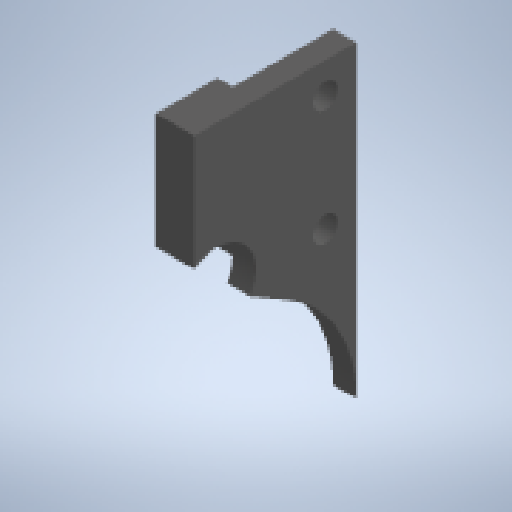
# Autodesk Inventor part: toe_springjoint_cover_upper_left
Saved by Autodesk Inventor 2024.1 (Build 281209000, 209)
## iProperties
Created: 2024-02-25
Part Number: toe_springjoint_cover_upper_left
Material: 一般
Document SubType Name: Modeling
Designer: hibik
Density: 1 g/cm^3
Appearance: 既定
Author: hibik
Autodesk Inventor part; units mm, degrees
ref_plane "YZ Plane" through (0, 0, 0) normal (1, 0, 0) x (0, 1, 0)
ref_plane "XZ Plane" through (0, 0, 0) normal (0, 1, 0) x (-1, 0, 0)
ref_plane "XY Plane" through (0, 0, 0) normal (0, 0, 1) x (1, 0, 0)
sketch "スケッチ1" plane through (0, 0, 0) normal (1, 0, 0) x (0, 1, 0)
  circle A0 centre (0, 0) radius 9
  line L0 (50, 5.5) -> (-9, 5.5)
  line L1 (-9, 5.5) -> (-9, -13.5)
  line L2 (-9, -13.5) -> (50, -13.5)
  line L3 (50, -13.5) -> (50, 5.5)
  line L4 (50, 13.5) -> (-9, 13.5)
  line L5 (-9, 13.5) -> (-9, -13.5)
  line L6 (-9, -13.5) -> (50, -13.5)
  line L7 (50, -13.5) -> (50, 13.5)
  line L8 (-20.8, 0) -> (61.8, 0) projected
  point P0 (-9, 0)
  dimension "d0" = 18
  dimension "d3" = 19
  dimension "d4" = 27
  constraints: 16 end point, 4 parallel, 2 horizontal, 2 perpendicular, 1 centre point, 1 coincident, 1 midpoint, 1 point on line, 1 tangent
  measures "d0" diameter of A0
  measures "d3" distance of L2.end L0.start
  measures "d4" distance of L4.end L1.end
extrude "押し出し1" add sketch "スケッチ1" along normal blind 1.5 contours L8 L3 L2 L1 A0 | A0 L0 L3 L8 | L1 L0 A0
sketch "スケッチ2" plane through (0, 0, 0) normal (-1, 0, 0) x (0, 0, 1)
  line L0 (1.5, 20) -> (1.5, 12.5) projected
  arc A0 (1.5, 12.5) -> (-2.1169, 9.1701) centre (0, 10.5) ccw projected
  line L1 (-2.1169, 9.1701) -> (-3.5, 8.3716) projected
  line L2 (-3.5, 8.3716) -> (-3.5, 20) projected
  line L3 (-3.5, 20) -> (1.5, 20) projected
  line L4 (-9, 20) -> (-3.5, 20) projected
  line L5 (-9, 0) -> (-9, 20) projected
  arc A1 (-4.5, 7.7942) -> (-9, 0) centre (0, 0) ccw projected
  line L6 (-3.5, 8.3716) -> (-4.5, 7.7942) projected
  arc A2 (5.5, 7.1239) -> (0, -9) centre (0, 0) ccw projected
  line L7 (5.5, 50) -> (5.5, 7.1239) projected
  line L8 (-13.5, 50) -> (5.5, 50) projected
  line L9 (-13.5, -9) -> (-13.5, 50) projected
  line L10 (0, -9) -> (-13.5, -9) projected
  line L11 (5.5, -9) -> (0, -9) projected
  line L12 (5.5, -7.1239) -> (5.5, -9) projected
  arc A3 (0, -9) -> (5.5, -7.1239) centre (0, 0) ccw projected
  point P0 (-4.5, 7.7942)
extrude "押し出し2" cut sketch "スケッチ2" against normal through all contours L3 L4 L5 A2 L10 L9 L8 L7 L6 L1 A0 L0 | A3 L12 L11
sketch "スケッチ3" plane through (0, 0, 0) normal (-1, 0, 0) x (0, 0, 1)
  line L0 (-3.5, 20) -> (-3.5, 8.3716) projected
  line L1 (-4.5, 7.7942) -> (-2.1169, 9.1701) projected
  arc A0 (1.5, 12.5) -> (-2.1169, 9.1701) centre (0, 10.5) ccw projected
  line L2 (1.5, 12.5) -> (1.5, 20) projected
  line L3 (1.5, 20) -> (-9, 20) projected
  line L4 (-9, 20) -> (-9, 0) projected
  arc A1 (-4.5, 7.7942) -> (-9, 0) centre (0, 0) ccw projected
  line L5 (-3.5, 20) -> (-2.5, 20)
  line L6 (-2.5, 20) -> (-2.5, 8.3716)
  line L7 (-2.5, 8.3716) -> (-3.5, 8.3716)
  line L8 (-3.5, 8.3716) -> (-3.5, 20)
  point P0 (-2.5, 10.5)
  dimension "d7" = 1
  constraints: 8 end point, 2 parallel, 1 horizontal, 1 perpendicular, 1 point on line
  measures "d7" distance between parallel lines of L6 L0
extrude "押し出し3" add sketch "スケッチ3" along normal blind 1 contours L3 L2 A0 L6
sketch "スケッチ4" plane through (1.5, 0, 0) normal (1, 0, 0) x (0, 0, -1)
  circle A0 centre (7, 18) radius 0.8
  circle A1 centre (7, 10.5) radius 0.8
  line L0 (9, 20) -> (-1.5, 20) projected
  line L1 (9, 0) -> (9, 20) projected
  arc A2 (2.1169, 9.1701) -> (-1.5, 12.5) centre (0, 10.5) ccw projected
  point P0 (0, 0)
  dimension "d10" = 1.6
  dimension "d11" = 1.6
  dimension "d12" = 2
  dimension "d13" = 2
  dimension "d14" = 2
  constraints: 2 centre point, 1 horizontal alignment
  measures "d10" diameter of A0
  measures "d11" diameter of A1
  measures "d12" distance from line of L0 A0.centre
  measures "d13" distance from line of L1 A0.centre
  measures "d14" distance from line of L1 A1.centre
extrude "押し出し4" cut sketch "スケッチ4" against normal through all
equation "\"d14\" = d13"
